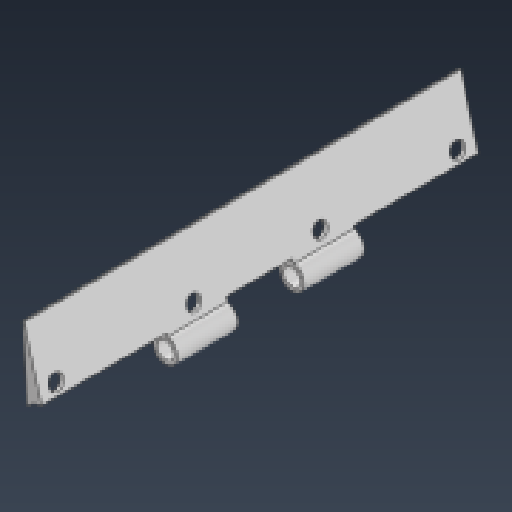
# Autodesk Inventor part: plug-hold
Saved by Autodesk Inventor 2023 (Build 270158000, 158)
## iProperties
Created: 2025-07-07
Part Number: plug-hold
Material: Generic
Document SubType Name: Modeling
Designer: szymo
Density: 1 g/cm^3
Appearance: Default
Author: szymo
Autodesk Inventor part; units mm, degrees
ref_plane "YZ Plane" through (0, 0, 0) normal (1, 0, 0) x (0, 1, 0)
ref_plane "XZ Plane" through (0, 0, 0) normal (0, 1, 0) x (-1, 0, 0)
ref_plane "XY Plane" through (0, 0, 0) normal (0, 0, 1) x (1, 0, 0)
ref_plane "Work Plane1" through (2, 5.1201, -5) normal (0, 0, 1) x (1, 0, 0)
sketch "Sketch1" plane through (2, 5.1201, -5) normal (0, 0, 1) x (1, 0, 0)
  circle A0 centre (1, -2.429) radius 1.7 projected
  line L0 (-2, -1.1863) -> (-1.1213, -0.3076) projected
  line L1 (-2, -5.1201) -> (-2, -1.1863) projected
  line L2 (-2, -5.1201) -> (0, -5.1201) projected
  line L3 (2.3258, -5.1201) -> (0, -5.1201) projected
  arc A1 (2.3258, -5.1201) -> (-1.1213, -0.3076) centre (1, -2.429) ccw projected
  line L4 (-5.7401, 22.7993) -> (-5.0833, 21.2085) projected
  line L5 (-5.7878, 22.7843) -> (-5.7401, 22.7993) projected
  line L6 (-5.7878, 22.7843) -> (-0.3953, 5.6111) projected
  line L7 (-0.3953, 5.6111) -> (-0.2045, 5.671) projected
  line L8 (-5.0833, 21.2085) -> (-0.2045, 5.671) projected
  line L9 (-2.0007, 6.0503) -> (-0.2032, 0.3259)
  line L10 (-2.0007, 6.0503) -> (-0.2455, 5.134)
  line L11 (-0.2032, 0.3259) -> (0.7131, 2.081)
  line L12 (-0.2455, 5.134) -> (0.7131, 2.081)
  circle A2 centre (1, -2.429) radius 2.8
  line L13 (-5.7878, 22.7843) -> (-5.7878, 4.3646)
  line L14 (-0.2455, 5.134) -> (-0.3953, 5.6111)
  line L15 (-4.2878, 18.0073) -> (-2, -1.1863)
  line L16 (0.7131, 2.081) -> (1.1891, 0.5651)
  line L17 (-4.0339, 15.8772) -> (-3.6339, 15.9248)
  line L18 (1.1891, 0.5651) -> (1.2537, 0.3595)
  line L19 (-2, -1.1863) -> (-1.7733, -2.815)
  circle A3 centre (1, -2.429) radius 1.9
  point P0 (3.4841, -1.1369)
  point P1 (-4.6303, 19.0981)
  point P2 (-1.7691, -2.8439)
  point P3 (0.2269, -5.1201)
  point P4 (1.7731, -5.1201)
  dimension "d1" = 6
  dimension "d2" = 45
  dimension "d3" = 45
  dimension "d7" = 5.6
  dimension "d51" = 0.5
  dimension "d52" = 3.2
  dimension "d53" = 1.5
  dimension "d54" = 0.4
  dimension "d88" = 0.2
  dimension "d89" = 0.9
  constraints: 22 end point, 7 point on line, 5 point on circle, 2 centre point, 1 coincident, 1 collinear, 1 perpendicular, 1 tangent, 1 vertical
  measures "d1" distance of L9.start L9.end
  measures "d2" angle of L9 L10
  measures "d3" angle of L9 L11
  measures "d7" diameter of A2
  measures "d51" distance of L10.end L6.end
  measures "d52" distance of L10.end L11.end
  measures "d53" distance from line of L13 L15.start
  measures "d54" horizontal distance of L17.start L17.end
  measures "d88" radial gap between concentric circles of A0 A3
  measures "d89" radial gap between concentric circles of A3 A2
ref_plane "Work Plane2" through (0, 0, -48.35) normal (0, 0, 1) x (1, 0, 0)
extrude "Extrusion1" add sketch "Sketch1" against normal up to surface (43.35 mm away) contours L15 L17 L6 L14 L10 L9 L11 L16 A1 L0 | L0 A1 L18 A2 L19 | A2 L3 | L3 A2 | L11 L9 L10 L12
sketch "Sketch2" plane through (2, 5.1201, -5) normal (0, 0, 1) x (1, 0, 0)
  arc A0 (-1.7733, -2.815) -> (1.2537, 0.3595) centre (1, -2.429) ccw projected
  line L0 (1.2537, 0.3595) -> (-3.6339, 15.9248) projected
  line L1 (-3.6339, 15.9248) -> (-4.0339, 15.8772) projected
  line L2 (-4.0339, 15.8772) -> (-2, -1.1863) projected
  line L3 (-2, -1.1863) -> (-1.7733, -2.815) projected
  circle A1 centre (1, -2.429) radius 1.7 projected
  circle A2 centre (1, -2.429) radius 2.8
  circle A3 centre (1, -2.429) radius 3.25
  line L4 (-1.6699, -0.5759) -> (-2.0671, -0.6232)
  line L5 (1.0756, 0.9264) -> (0.694, 0.8066)
  point P0 (-1.5871, -1.3581)
  point P1 (1.214, 0.4858)
  point P2 (0.8324, 0.366)
  dimension "d57" = 0.4
  dimension "d58" = 6.5
  dimension "d59" = 90
  dimension "d60" = 90
  dimension "d62" = 0.4
  dimension "d63" = 0.4
  constraints: 5 point on circle, 4 end point, 3 point on line, 2 centre point, 2 coincident
  measures "d57" distance of point (1.214, 0.486) point (0.832, 0.366)
  measures "d58" diameter of A3
  measures "d59" angle of L0 L5
  measures "d60" angle of L2 L4
  measures "d62" distance of L5.start L5.end
  measures "d63" distance of L4.start L4.end
ref_plane "Work Plane3" through (0, -39.3088, 22.825) normal (0, 0, 1) x (1, 0, 0)
extrude "Extrusion2" add sketch "Sketch2" along normal blind 27.825 and the other way blind 71.175 contours L2 L1 L0 L5 A3 L4
sketch "Sketch3" plane through (0.1975, 2.2765, -48.35) normal (-0.9929711, -0.1183574, 0) x (0, 0, 1)
  line L0 (41.05, -61.835) -> (4.45, -61.835) projected
  line L1 (4.45, -61.835) -> (4.45, -46.083) projected
  ellipse E0 centre (8.45, -46.083) end of major axis (4.45, -46.083) minor radius 3.9968 (8.45, -42.0862) -> (4.45, -46.083) ccw projected
  line L2 (8.45, -42.0862) -> (41.05, -42.0862) projected
  ellipse E1 centre (41.05, -46.083) end of major axis (37.05, -46.083) minor radius 3.9968 (45.05, -46.083) -> (41.05, -42.0862) ccw projected
  line L3 (45.05, -46.083) -> (45.05, -57.8382) projected
  ellipse E2 centre (41.05, -57.8382) end of major axis (45.05, -57.8382) minor radius 3.9968 (41.05, -61.835) -> (45.05, -57.8382) ccw projected
  ellipse E3 centre (0.8602, -63.4008) end of major axis (4.3602, -63.4008) minor radius 3.4972 projected
  ellipse E4 centre (44.1757, -80.3152) end of major axis (47.6757, -80.3152) minor radius 3.4972 projected
  ellipse E5 centre (43.084, -68.4892) end of major axis (46.584, -68.4892) minor radius 3.4972 projected
  ellipse E6 centre (-0.1912, -46.1212) end of major axis (3.3088, -46.1212) minor radius 3.4972 projected
  line L4 (43.35, 1.1221) -> (43.35, -2.8086) projected
  line L5 (43.35, -2.8086) -> (28.675, -2.8086) projected
  line L6 (28.675, -2.8086) -> (28.675, 1.1221) projected
  line L7 (28.675, 1.1221) -> (14.675, 1.1221) projected
  line L8 (14.675, 1.1221) -> (14.675, -2.8086) projected
  line L9 (14.675, -2.8086) -> (0, -2.8086) projected
  line L10 (0, -2.8086) -> (0, 1.1221) projected
  line L11 (0, 1.1221) -> (-5, 1.1221) projected
  line L12 (-5, 1.1221) -> (-5, -2.8086) projected
  line L13 (-5, -2.8086) -> (-9, -2.8086) projected
  line L14 (-9, -17.2527) -> (-9, -2.8086) projected
  line L15 (-21.1707, -17.2527) -> (-9, -17.2527) projected
  ellipse E7 centre (-24.075, -19.2044) end of major axis (-20.575, -19.2044) minor radius 3.4972 (-26.9793, -17.2527) -> (-21.1707, -17.2527) ccw projected
  line L16 (-27.825, -17.2527) -> (-26.9793, -17.2527) projected
  line L17 (-27.825, -42.0862) -> (-27.825, -17.2527) projected
  line L18 (-27.825, -42.0862) -> (-24.075, -42.0862) projected
  ellipse E8 centre (-24.075, -38.589) end of major axis (-20.575, -38.589) minor radius 3.4972 projected
  line L19 (-24.075, -42.0862) -> (-8.35, -42.0862) projected
  line L20 (-8.35, -42.0862) -> (-8.35, -85.9539) projected
  line L21 (-8.35, -85.9539) -> (-1.7, -85.9539) projected
  line L22 (-1.7, -85.9539) -> (-1.7, -78.6925) projected
  ellipse E9 centre (2.3, -78.6925) end of major axis (-1.7, -78.6925) minor radius 3.9968 (2.3, -74.6957) -> (-1.7, -78.6925) ccw projected
  line L23 (2.3, -74.6957) -> (38.9, -74.6957) projected
  line L24 (38.9, -74.6957) -> (38.9, -85.9539) projected
  line L25 (38.9, -85.9539) -> (51.7, -85.9539) projected
  line L26 (51.7, -85.9539) -> (51.7, -42.0862) projected
  line L27 (51.7, -42.0862) -> (67.425, -42.0862) projected
  ellipse E10 centre (67.425, -38.589) end of major axis (70.925, -38.589) minor radius 3.4972 projected
  line L28 (67.425, -42.0862) -> (71.175, -42.0862) projected
  line L29 (71.175, -17.2527) -> (71.175, -42.0862) projected
  line L30 (70.3293, -17.2527) -> (71.175, -17.2527) projected
  ellipse E11 centre (67.425, -19.2044) end of major axis (70.925, -19.2044) minor radius 3.4972 (64.5207, -17.2527) -> (70.3293, -17.2527) ccw projected
  line L31 (52.35, -17.2527) -> (64.5207, -17.2527) projected
  line L32 (52.35, -2.8086) -> (52.35, -17.2527) projected
  line L33 (52.35, -2.8086) -> (48.35, -2.8086) projected
  line L34 (48.35, -2.2371) -> (48.35, 1.1221) projected
  line L35 (48.35, 1.1221) -> (43.35, 1.1221) projected
  line L36 (-27.825, 7.6648) -> (0, 7.6648) projected
  line L37 (43.35, 7.6648) -> (71.175, 7.6648) projected
  line L38 (0, 7.6648) -> (43.35, 7.6648)
  line L39 (43.35, -2.7199) -> (0, -2.7199) projected
  line L40 (0.5, -2.7199) -> (0.5, 7.6648)
  line L41 (14.175, -2.7199) -> (14.175, 7.6648)
  line L42 (29.175, -2.7199) -> (29.175, 7.6648)
  line L43 (42.85, 7.6648) -> (42.85, -2.7199)
  line L44 (43.35, 1.1221) -> (43.35, 7.6648)
  line L45 (43.35, 1.9344) -> (43.35, -1.4656) projected
  line L46 (0, 1.1221) -> (0, 7.6648)
  line L47 (0, -1.4656) -> (0, 1.9344) projected
  line L48 (43.35, 2.2362) -> (71.175, 2.2362) projected
  line L49 (-27.825, 2.2362) -> (0, 2.2362) projected
  line L50 (43.35, 2.2362) -> (43.35, 1.6691) projected
  line L51 (0, 2.2362) -> (43.35, 2.2362)
  point P0 (0.5, 2.2362)
  point P1 (29.175, 2.2362)
  point P2 (14.175, 2.2362)
  point P3 (42.85, 2.2362)
  dimension "d16" = 0.5
  dimension "d17" = 0.5
  dimension "d18" = 0.5
  dimension "d19" = 0.5
  constraints: 16 end point, 8 point on line, 4 perpendicular, 2 collinear, 2 vertical alignment, 1 parallel, 6 other
  measures "d16" distance between parallel lines of L40 L10
  measures "d17" distance between parallel lines of L41 L8
  measures "d18" distance between parallel lines of L42 L6
  measures "d19" distance between parallel lines of L43 L4
extrude "Extrusion3" cut sketch "Sketch3" against normal blind 27.825 contours L4 L39 L43 L51 L44 | L39 L6 L7 L8 L41 L51 L42 | L39 L8 L7 L6 | L40 L39 L10 L46 L51
sketch "Sketch4" plane through (1.9471, 10.7832, -5) normal (0, 0, 1) x (0.9510489, 0.3090404, 0)
  line L0 (-3.466, -5.4338) -> (0.6719, -6.2534) projected
  arc A0 (0.6719, -6.2534) -> (-0.3964, -5.4477) centre (-1.4994, -8.0213) ccw projected
  line L1 (-0.3964, -5.4477) -> (-0.3905, -4.8535) projected
  line L2 (-0.3905, -4.8535) -> (-0.7905, -4.8495) projected
  arc A1 (-0.7905, -4.8495) -> (-3.466, -5.4338) centre (-1.4994, -8.0213) ccw projected
extrude "Extrusion4" cut sketch "Sketch4" against normal up to surface (0.5 mm away)
sketch "Sketch9" plane through (4.5187, 5.0435, -48.35) normal (0, 0, -1) x (-0.9929711, -0.1183574, 0)
  line L0 (0, 0) -> (4.2183, 0) projected
  arc A0 (4.2183, 0) -> (1.7073, 1.093) centre (1.7864, -2.1561) ccw projected
  line L1 (1.7073, 1.093) -> (1.3142, 1.1668) projected
  line L2 (1.3142, 1.1668) -> (1.2045, 0.5828) projected
  arc A1 (1.2045, 0.5828) -> (0, 0) centre (1.7864, -2.1561) ccw projected
  point P0 (5.0839, -4.4732)
extrude "Extrusion8" cut sketch "Sketch9" against normal up to surface (0.5 mm away)
ref_plane "Work Plane4" through (-0.0671, 4.4969, -76.175) normal (0.954071, 0.2995806, 0) x (0, 0, -1)
sketch "Sketch10" plane through (-0.0671, 4.4969, -76.175) normal (0.954071, 0.2995806, 0) x (0, 0, -1)
  line L0 (-28.325, 0.537) -> (0, 0.537) projected
  line L1 (0, 16.2574) -> (0, 0.537) projected
  line L2 (0, 16.2574) -> (-99, 16.2574) projected
  line L3 (-99, 0.537) -> (-99, 16.2574) projected
  line L4 (-99, 0.537) -> (-70.675, 0.537) projected
  line L5 (-70.675, 0.537) -> (-70.675, -0.0572) projected
  line L6 (-70.675, -0.0572) -> (-28.325, -0.0572) projected
  line L7 (-28.325, -0.0572) -> (-28.325, 0.537) projected
  line L8 (0, 0) -> (-28.325, 0) projected
  line L9 (-28.325, 0) -> (-28.325, -0.5574) projected
  line L10 (-42, -0.5574) -> (-28.325, -0.5574) projected
  line L11 (-42, -0.5574) -> (-42, 0) projected
  line L12 (-42, 0) -> (-57, 0) projected
  line L13 (-57, 0) -> (-57, -0.5574) projected
  line L14 (-70.675, -0.5574) -> (-57, -0.5574) projected
  line L15 (-70.675, -0.5574) -> (-70.675, 0) projected
  line L16 (-70.675, 0) -> (-99, 0) projected
  line L17 (-99, 16.3317) -> (-99, 0) projected
  line L18 (-99, 16.3317) -> (0, 16.3317) projected
  line L19 (0, 0) -> (0, 16.3317) projected
  line L20 (-99, 0) -> (-91, 0)
  line L21 (-91, 0) -> (-91, 6)
  line L22 (-91, 6) -> (-99, 6)
  line L23 (-99, 6) -> (-99, 0)
  line L24 (0, 0) -> (-8, 0)
  line L25 (-8, 0) -> (-8, 6)
  line L26 (-8, 6) -> (0, 6)
  line L27 (0, 6) -> (0, 0)
  line L28 (-70.675, 0) -> (-28.325, 0)
  line L29 (-38.1625, 0) -> (-32.1625, 0)
  line L30 (-32.1625, 0) -> (-32.1625, 6)
  line L31 (-32.1625, 6) -> (-38.1625, 6)
  line L32 (-38.1625, 6) -> (-38.1625, 0)
  line L33 (-66.8375, 0) -> (-60.8375, 0)
  line L34 (-60.8375, 0) -> (-60.8375, 6)
  line L35 (-60.8375, 6) -> (-66.8375, 6)
  line L36 (-66.8375, 6) -> (-66.8375, 0)
  line L37 (-38.1625, 0) -> (-32.1625, 6)
  line L38 (-32.1625, 0) -> (-38.1625, 6)
  line L39 (-8, 6) -> (0, 0)
  line L40 (-8, 0) -> (0, 6)
  line L41 (-91, 0) -> (-99, 6)
  line L42 (-99, 0) -> (-91, 6)
  line L43 (-66.8375, 0) -> (-60.8375, 6)
  line L44 (-66.8375, 6) -> (-60.8375, 0)
  point P0 (-76.175, -4.3105)
  point P1 (-95, 3)
  point P2 (-63.8375, 3)
  point P3 (-35.1625, 3)
  point P4 (-4, 3)
  dimension "d66" = 8
  dimension "d67" = 6
  dimension "d68" = 8
  dimension "d69" = 6
  dimension "d70" = 6
  dimension "d71" = 6
  dimension "d72" = 6
  dimension "d73" = 6
  dimension "d75" = 3.8375
  dimension "d76" = 3.8375
  dimension "d77" = 3.8375
  dimension "d78" = 3.8375
  constraints: 50 end point, 9 parallel, 5 midpoint, 4 horizontal, 4 perpendicular, 2 point on line
  measures "d66" distance of L22.end L21.end
  measures "d67" distance of L21.end L20.end
  measures "d68" distance of L25.end L26.end
  measures "d69" distance of L24.end L25.end
  measures "d70" distance of L31.end L30.end
  measures "d71" distance of L30.end L29.end
  measures "d72" distance of L35.end L34.end
  measures "d73" distance of L34.end L33.end
  measures "d75" distance between parallel lines of L34 L13
  measures "d76" distance between parallel lines of L36 L15
  measures "d77" distance between parallel lines of L32 L11
  measures "d78" distance between parallel lines of L30 L9
hole "Hole2" at (-0.9659, 7.3591, 18.825) at (-0.9659, 7.3591, -12.3375) at (-0.9659, 7.3591, -41.0125) at (-0.9659, 7.3591, -72.175) direction (0.954071, 0.2995806, 0) diameter 3.4 end through all countersink diameter 8.5 countersink angle 90 clearance for "Countersunk Flat Head Screw ISO 2009/7046" size "M3" standard "ISO"
sketch "Sketch11" plane through (0, 3.9338, -34.175) normal (0, 0, 1) x (0.9929711, 0.1183574, 0)
  arc A0 (0.0324, -1.6441) -> (3.4138, 1.1499) centre (2.8318, -1.589) ccw projected
  line L0 (0, 0.5671) -> (0.4, 0.5671) projected
  line L1 (0, 0) -> (0, 0.5671) projected
  line L2 (0.0324, -1.6441) -> (0, 0) projected
  line L3 (3.3041, 1.7339) -> (3.4138, 1.1499) projected
  line L4 (3.3041, 1.7339) -> (2.911, 1.6601) projected
  arc A1 (2.911, 1.6601) -> (0.4, 0.5671) centre (2.8318, -1.589) ccw projected
  point P0 (-0.4656, -3.9061)
extrude "Extrusion9" cut sketch "Sketch11" along normal up to surface (15 mm away)
sketch "Sketch12" plane through (0, 3.9338, -34.175) normal (0, 0, 1) x (0.9929711, 0.1183574, 0)
  arc A0 (5.2726, -3.3333) -> (0.3555, 0.1044) centre (2.8318, -1.589) ccw projected
  circle A1 centre (2.8318, -1.589) radius 3.7
  circle A2 centre (2.8318, -1.589) radius 1.9 projected
  arc A3 (0.0324, -1.6441) -> (3.4138, 1.1499) centre (2.8318, -1.589) ccw projected
  line L0 (3.3041, 1.7339) -> (3.4138, 1.1499) projected
  line L1 (3.3041, 1.7339) -> (2.911, 1.6601) projected
  arc A4 (2.911, 1.6601) -> (0.4, 0.5671) centre (2.8318, -1.589) ccw projected
  line L2 (0, 0.5671) -> (0.4, 0.5671) projected
  line L3 (0, 0) -> (0, 0.5671) projected
  line L4 (0.0324, -1.6441) -> (0, 0) projected
  line L5 (0, 17.1843) -> (0, 0.5671) projected
  line L6 (0, 0.5671) -> (0.4, 0.5671) projected
  arc A5 (2.911, 1.6601) -> (0.4, 0.5671) centre (2.8318, -1.589) ccw projected
  line L7 (2.911, 1.6601) -> (3.3041, 1.7339) projected
  line L8 (3.3041, 1.7339) -> (0.4028, 17.1843) projected
  line L9 (0.4028, 17.1843) -> (0, 17.1843) projected
  line L10 (0.4028, 17.1843) -> (3.3041, 1.7339) projected
  line L11 (3.2192, 2.1861) -> (2.8192, 2.111)
  line L12 (0.4, 1.1996) -> (0, 1.1996)
  line L13 (0, 0.5671) -> (0, 17.1843) projected
  point P0 (-0.4656, -3.9061)
  point P1 (3.3041, 1.7339)
  point P2 (3.2375, 2.0887)
  point P3 (0.0841, 0.6262)
  point P4 (0, 0.7923)
  point P5 (0, 0.5671)
  dimension "d90" = 7.4
  dimension "d91" = 0.4
  dimension "d92" = 0.4
  constraints: 4 end point, 2 perpendicular, 2 point on circle, 2 point on line, 1 centre point, 1 coincident
  measures "d90" diameter of A1
  measures "d91" horizontal distance of L11.start L11.end
  measures "d92" distance of L12.start L12.end
extrude "Extrusion10" cut sketch "Sketch12" along normal up to surface (15 mm away) contours A1 L8 L1 A4 L2 L5 | A1 L5 L3 L4 A3 L0 L8 | L0 A3 L4 L3 L2 A4 L1 | A2
equation "\"d17\" = d16"
equation "\"d18\" = d16"
equation "\"d19\" = d16"
equation "\"d76\" = d75"
equation "\"d77\" = d78"
body "Solid1"
